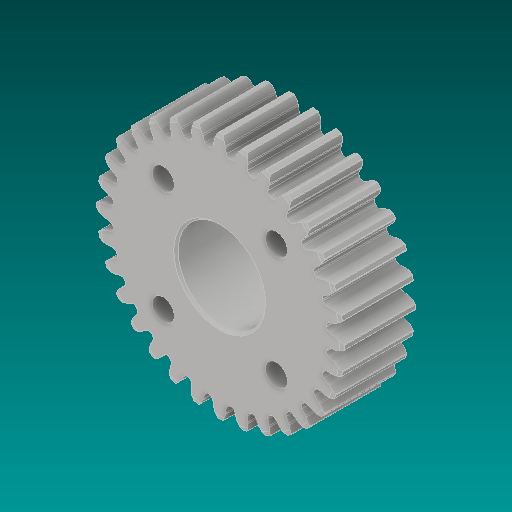
# Autodesk Inventor part: GEABP1.0-32-10-A-12-KFC22-K3_b
Saved by Autodesk Inventor 2020 (Build 240168000, 168)
## iProperties
Created: 2022-11-01
Part Number: GEABP1.0-32-10-A-12-KFC22-K3_b
Material: Generic
Catalog Web Link: www.cadenas.de
Description: GEABM, GEABMS, GEABMT, GEABP, GEABPS, GEABPT, GEABA, GEABAS, GEABAT_body-Plastic Spur Gears - Pressure Angle 20 Degrees, Module 0.5/0.8/1.0/1.5/2.0/2.5/3.0
Vendor: MISUMI
Document SubType Name: Modeling
Designer: psAdmin
Manufacturer: MISUMI
Mass: 6.51664 g
Surface Area: 40.015 cm^2
Volume: 6.51664 cm^3
Density: 1 g/cm^3
Appearance: PSOLRGB-175-175-175
Category: PARTsolutions
Company: MISUMI
PSOL_IDENT_0: {$CADENAS_DATA/23d-libs/misumi/metric/54_spur_gears/geabms20/geabms20.prj},408 {VTYP=3D},{NB=GEABP1.
PSOL_IDENT_1: 0-32-10-A-12-KFC22-K3_b},{LINA=GEABP1.0-32-10-A-12-KFC22-K3},{NN=GEABM, GEABMS, GEABMT, GEABP, GEABP
PSOL_IDENT_2: S, GEABPT, GEABA, GEABAS, GEABAT_body},{DATE=17.10.2022 23:48:33},{GEOMDATE=14.09.2022 05:11:00},{VE
PSOL_IDENT_3: RSION=},{LINEID=30},{WBVAR=MATSG,MATCR,NT,B,TS,PS,ALT1,ALT2,TPC,ALT11,ALT10,BS,ALT3,Z,J,ALT4,Q,R,S,T
PSOL_IDENT_4: ,ALT5,LFC,LTC,MALT5,ALT6,KFC,KTC,K},{WBNUMERIC=NT,B,BS,Z,J,Q,R,S,T,LFC,LTC,KFC,KTC,K}  {NB=GEABP1.0-
PSOL_IDENT_5: 32-10-A-12-KFC22-K3_b},{LINA=GEABP1.0-32-10-A-12-KFC22-K3},{KT=DUMMY},{PN=GEABP1.0-32-10-A-12-KFC22-
PSOL_IDENT_6: K3},{TYPE=GEABP},{MATSG=PW},{MATSGALG='MCN','MC Nylon','PW','Polyacetal White','PB','Polyacetal Blue'
PSOL_IDENT_7: },{MATCR=},{MATCRALG='','-','S45C','1045 Carbon Steel','SUS304','304 Stainless Steel'},{MOD=1.0},{MO
PSOL_IDENT_8: D1=1.0},{NT=32},{NTALG=15,16,18,20,22,24,25,26,28,30,32,35,36,40,45,48,50,55,60,70,75,80,90,100,120}
PSOL_IDENT_9: ,{B=10},{BALG=10,15},{TS=A},{TSALG='A','A','B','B'},{TSPN=-A},{PS=12},{PSALG='10','10','11','11','12'
PSOL_IDENT_10: ,'12','13','13','14','14','15','15','16','16','17','17','18','18'},{PSCRL='10','10','11','11','12','
PSOL_IDENT_11: 12','13','13','14','14','15','15','16','16','17','17','18','18'},{PSCRW='10','10','12','12'},{DD=32.
PSOL_IDENT_12: 0},{DD05=16},{DD08=25.6},{DD10=32},{DD15=48},{DD20=64},{DD25=80},{DD30=96},{D=34.0},{D05=17},{D08=27
PSOL_IDENT_13: .2},{D10=34},{D15=51},{D20=68},{D25=85},{D30=102},{G=29.50},{G05=14.75},{G08=23.6},{G10=29.5},{G15=4
PSOL_IDENT_14: 4.25},{G20=59},{G25=73.75},{G30=88.5},{H=0.0},{L=0},{LL1=0},{LL2=0.0},{M=-},{M3D=0},{P=12.00},{DD1=0
PSOL_IDENT_15: },{CIFR=15},{CIFM=0},{CIFK=0},{CIFTAP=0},{ALT1=},{ALT1ALG='','Not applicable'},{ALT1PN=},{ALT2=},{AL
PSOL_IDENT_16: T2ALG='','Not applicable'},{TPC=N/A},{TPCALG='N/A'},{ALT2PN=},{KC=0},{ALT11=},{ALT11ALG='','Not appl
PSOL_IDENT_17: icable'},{ALT11PN=},{DEG=0},{ALT10=},{ALT10ALG= '','Not applicable' },{ALT10PN=},{BS=0.0},{BSALG=0},
PSOL_IDENT_18: {BSMIN=3},{BSMINALG=3.000},{BSMAX=0},{LL13D=0},{LL23D=0},{LBS=10},{ALT3=},{ALT3ALG= '','w/o Stepped
PSOL_IDENT_19: Hole','DHL','with DHL (Stepped Hole)','DHR','with DHR (Stepped Hole)' },{ALT3PN=},{ZJPN=},{ALT31=1},
PSOL_IDENT_20: {ALT32=1},{Z=0},{ZALG=0},{ZMINL=14},{ZMAXL=25},{ZMINR=14},{ZMAXR=25},{ZPN=},{J=0.0},{JALG=0},{JMIN=2
PSOL_IDENT_21: },{JMAX=0},{JPN=},{ALT4=},{ALT4ALG= '','w/o WDH (Both Ends Stepped Hole)','WDH','with WDH (Both Ends
PSOL_IDENT_22: Stepped Hole)' },{ALT4PN=},{QRSTPN=},{LB=10.000},{Q=0},{QALG=0},{QMIN=14},{QMAX=25},{QPN=},{R=0},{R
PSOL_IDENT_23: ALG=0},{RMIN=14},{RMAX=25},{RPN=},{S=0},{SALG=0},{SMIN=3},{SMAX=4},{SPN=},{T=0},{TALG=0},{TMIN=3},{T
PSOL_IDENT_24: MAX=0},{TPN=},{ALT5=},{ALT5ALG= '','w/o Side Slotted Hole','LFC','with LFC (Side Slotted Hole)','LTC'
PSOL_IDENT_25: ,'with LTC (Side Slotted Hole)' },{LFC=0},{LFCALG=0},{LTC=0},{LTCALG=0},{LPCDMIN=20},{LPCDMAX=22},{L
PSOL_IDENT_26: CMAX=25},{MALT5=N/A},{MALT5ALG= 'N/A' },{LCMAX2=22},{C=0.0},{ALT5PN=},{ALT6=KFC},{ALT6ALG= '','w/o S
PSOL_IDENT_27: ide Through Hole','KFC','with KFC (Side Through Hole)','KTC','with KTC (Side Through Hole)' },{ALT6P
PSOL_IDENT_28: N=-KFC},{KFTCPN=22-K3},{KFC=22},{KFCALG=[19:22/1]},{KFCPN=22},{KTC=0},{KTCALG=[0]},{KTCPN=},{KPCDMIN
PSOL_IDENT_29: 1=19},{KPCDMAX1=-7},{KPCDMIN2=7},{KPCDMAX2=22},{K=3.0},{KALG=[3:3.5/0.5]},{KPCD=22},{KPN=-K3},{SCREW=
PSOL_IDENT_30: 0},{SCREWL=0},{AG=0},{PCD=22},{SHN=4},{SHDEG1=45},{SHDEG2=90},{PZQRDD2=12},{D1=2.8125},{D2=5.625},{D
PSOL_IDENT_31: 3=20},{D4=0.1},{D5=5.333333},{D6=4.923077},{D7=0.85},{D8=0.5},{D9=0.821781},{S1=15},{S2=0.5},{KR=15}
NB: GEABP1.0-32-10-A-12-KFC22-K3_b
NN: GEABM, GEABMS, GEABMT, GEABP, GEABPS, GEABPT, GEABA, GEABAS, GEABAT_body
NT: 32
NBSYN: $PN._b
LINA: GEABP1.0-32-10-A-12-KFC22-K3
CATALOG: Misumi
PN: GEABP1.0-32-10-A-12-KFC22-K3
MATSG: Polyacetal White
MATCR: -
MOD: 1.0
B: 10
TS: A
PS: 12
DD: 32
D: 34
G: 29.5
H: 0
L: 0
LL1: 0
LL2: 0
M: -
DD1: 0
ALT1: Not applicable
ALT2: Not applicable
TPC: N/A
ALT11: Not applicable
ALT10: Not applicable
BS: 0
ALT3: w/o Stepped Hole
Z: 0
J: 0
ALT4: w/o WDH (Both Ends Stepped Hole)
Q: 0
R: 0
S: 0
T: 0
ALT5: w/o Side Slotted Hole
LFC: 0
LTC: 0
MALT5: N/A
C: 0
ALT6: with KFC (Side Through Hole)
KFC: 22
KTC: 0
K: 3
SUPPLIER: MISUMI
ARTICLENO: GEABP1.0-32-10-A-12-KFC22-K3_b
BOMINFO: GEABP1.0-32-10-A-12-KFC22-K3
CREATOR: CADENAS GmbH
Title: GEABP1.0-32-10-A-12-KFC22-K3
Author: Cadenas PARTsolutions
Comments: Plastic Spur Gears - Pressure Angle 20 Degrees, Module 0.5/0.8/1.0/1.5/2.0/2.5/3.0
Autodesk Inventor part; units mm, degrees
ref_plane "YZ Plane" through (0, 0, 0) normal (1, 0, 0) x (0, 1, 0)
ref_plane "XZ Plane" through (0, 0, 0) normal (0, 1, 0) x (-1, 0, 0)
ref_plane "XY Plane" through (0, 0, 0) normal (0, 0, 1) x (1, 0, 0)
sketch "_____3" plane through (0, 0, 0) normal (1, 0, 0) x (0, 0, -1)
  line L0 (10, 0) -> (0, 0)
  line L1 (0, 0) -> (0, 16.5)
  line L2 (0, 16.5) -> (0.6699, 19)
  line L3 (0.6699, 19) -> (9.3301, 19)
  line L4 (9.3301, 19) -> (10, 16.5)
  line L5 (10, 16.5) -> (10, 0)
  line L6 (10, 0) -> (0, 0)
  constraints: 14 end point
revolve "Revolution1" add sketch "_____3" angle 360 about axis through (0, 0, -10) along (0, 0, -1)
sketch "_____12" plane through (0, 0, 0) normal (0, 0, 1) x (1, 0, 0)
  circle A0 centre (0, 0) radius 68
  arc A1 (-16.9975, 0.2932) -> (-16.9975, -0.2932) centre (0, 0) ccw
  arc A2 (-16.9975, -0.2932) -> (-16.9451, -0.3794) centre (-16.8975, -0.2914) ccw
  arc A3 (-16.9451, -0.3794) -> (-15.9807, -0.7851) centre (-14.4047, 4.3101) ccw
  arc A4 (-15.9807, -0.7851) -> (-15.7971, -0.8196) centre (-15.7379, 0) ccw
  arc A5 (-15.0745, -0.9267) -> (-15.7971, -0.8196) centre (-16.1556, -5.7297) ccw
  arc A6 (-14.6864, -1.3682) -> (-15.0745, -0.9267) centre (-15.1843, -1.4145) ccw
  arc A7 (-14.6864, -1.3682) -> (-14.6711, -1.5233) centre (0, 0) ccw
  arc A8 (-14.9656, -2.0319) -> (-14.6711, -1.5233) centre (-15.1685, -1.5749) ccw
  arc A9 (-15.6535, -2.278) -> (-14.9656, -2.0319) centre (-16.9629, 2.4678) ccw
  arc A10 (-15.6535, -2.278) -> (-15.8268, -2.3477) centre (-15.4355, -3.0703) ccw
  arc A11 (-15.8268, -2.3477) -> (-16.6935, -2.9338) centre (-13.2871, -7.0375) ccw
  arc A12 (-16.6935, -2.9338) -> (-16.7281, -3.0285) centre (-16.6297, -3.0107) ccw
  arc A13 (-16.7281, -3.0285) -> (-16.6137, -3.6036) centre (0, 0) ccw
  arc A14 (-16.6137, -3.6036) -> (-16.5455, -3.6779) centre (-16.516, -3.5824) ccw
  arc A15 (-16.5455, -3.6779) -> (-15.5205, -3.8877) centre (-14.9688, 1.417) ccw
  arc A16 (-15.5205, -3.8877) -> (-15.3337, -3.8858) centre (-15.4355, -3.0703) ccw
  arc A17 (-14.604, -3.8498) -> (-15.3337, -3.8858) centre (-14.7273, -8.7714) ccw
  arc A18 (-14.1373, -4.2071) -> (-14.604, -3.8498) centre (-14.6165, -4.3497) ccw
  arc A19 (-14.1373, -4.2071) -> (-14.092, -4.3562) centre (0, 0) ccw
  arc A20 (-14.2816, -4.9125) -> (-14.092, -4.3562) centre (-14.5697, -4.5039) ccw
  arc A21 (-14.9083, -5.288) -> (-14.2816, -4.9125) centre (-17.1184, -0.889) ccw
  arc A22 (-14.9083, -5.288) -> (-15.0647, -5.3902) centre (-14.5399, -6.0226) ccw
  arc A23 (-15.0647, -5.3902) -> (-15.8004, -6.1341) centre (-11.6588, -9.4944) ccw
  arc A24 (-15.8004, -6.1341) -> (-15.8158, -6.2338) centre (-15.7228, -6.1971) ccw
  arc A25 (-15.8158, -6.2338) -> (-15.5914, -6.7755) centre (0, 0) ccw
  arc A26 (-15.5914, -6.7755) -> (-15.5101, -6.8351) centre (-15.4997, -6.7356) ccw
  arc A27 (-15.5101, -6.8351) -> (-14.4638, -6.8409) centre (-14.9576, -1.5305) ccw
  arc A28 (-14.4638, -6.8409) -> (-14.281, -6.8025) centre (-14.5399, -6.0226) ccw
  arc A29 (-13.5723, -6.6249) -> (-14.281, -6.8025) centre (-12.7331, -11.476) ccw
  arc A30 (-13.0449, -6.8843) -> (-13.5723, -6.6249) centre (-13.4871, -7.1176) ccw
  arc A31 (-13.0449, -6.8843) -> (-12.9714, -7.0217) centre (0, 0) ccw
  arc A32 (-13.0488, -7.6044) -> (-12.9714, -7.0217) centre (-13.4111, -7.2598) ccw
  arc A33 (-13.5902, -8.0949) -> (-13.0488, -7.6044) centre (-16.6161, -4.2115) ccw
  arc A34 (-13.5902, -8.0949) -> (-13.7237, -8.2256) centre (-13.0856, -8.7435) ccw
  arc A35 (-13.7237, -8.2256) -> (-14.3001, -9.0988) centre (-9.5825, -11.5865) ccw
  arc A36 (-14.3001, -9.0988) -> (-14.2958, -9.1995) centre (-14.2117, -9.1454) ccw
  arc A37 (-14.2958, -9.1995) -> (-13.97, -9.687) centre (0, 0) ccw
  arc A38 (-13.97, -9.687) -> (-13.8786, -9.7296) centre (-13.8878, -9.6301) ccw
  arc A39 (-13.8786, -9.7296) -> (-12.8513, -9.5312) centre (-14.3716, -4.4191) ccw
  arc A40 (-12.8513, -9.5312) -> (-12.6795, -9.4579) centre (-13.0856, -8.7435) ccw
  arc A41 (-12.0191, -9.1455) -> (-12.6795, -9.4579) centre (-10.2496, -13.7396) ccw
  arc A42 (-11.4512, -9.2969) -> (-12.0191, -9.1455) centre (-11.8394, -9.6121) ccw
  arc A43 (-11.4512, -9.2969) -> (-11.3523, -9.4174) centre (0, 0) ccw
  arc A44 (-11.3146, -10.0039) -> (-11.3523, -9.4174) centre (-11.7371, -9.7367) ccw
  arc A45 (-11.7498, -10.5907) -> (-11.3146, -10.0039) centre (-15.4752, -7.3722) ccw
  arc A46 (-11.7498, -10.5907) -> (-11.8552, -10.7449) centre (-11.1284, -11.1284) ccw
  arc A47 (-11.8552, -10.7449) -> (-12.2503, -11.7138) centre (-7.138, -13.2334) ccw
  arc A48 (-12.2503, -11.7138) -> (-12.2263, -11.8117) centre (-12.1544, -11.7423) ccw
  arc A49 (-12.2263, -11.8117) -> (-11.8117, -12.2263) centre (0, 0) ccw
  arc A50 (-11.8117, -12.2263) -> (-11.7138, -12.2503) centre (-11.7423, -12.1544) ccw
  arc A51 (-11.7138, -12.2503) -> (-10.7449, -11.8552) centre (-13.2334, -7.138) ccw
  arc A52 (-10.7449, -11.8552) -> (-10.5907, -11.7498) centre (-11.1284, -11.1284) ccw
  arc A53 (-10.0039, -11.3146) -> (-10.5907, -11.7498) centre (-7.3722, -15.4752) ccw
  arc A54 (-9.4174, -11.3523) -> (-10.0039, -11.3146) centre (-9.7367, -11.7371) ccw
  arc A55 (-9.4174, -11.3523) -> (-9.2969, -11.4512) centre (0, 0) ccw
  arc A56 (-9.1455, -12.0191) -> (-9.2969, -11.4512) centre (-9.6121, -11.8394) ccw
  arc A57 (-9.4579, -12.6795) -> (-9.1455, -12.0191) centre (-13.7396, -10.2496) ccw
  arc A58 (-9.4579, -12.6795) -> (-9.5312, -12.8513) centre (-8.7435, -13.0856) ccw
  arc A59 (-9.5312, -12.8513) -> (-9.7296, -13.8786) centre (-4.4191, -14.3716) ccw
  arc A60 (-9.7296, -13.8786) -> (-9.687, -13.97) centre (-9.6301, -13.8878) ccw
  arc A61 (-9.687, -13.97) -> (-9.1995, -14.2958) centre (0, 0) ccw
  arc A62 (-9.1995, -14.2958) -> (-9.0988, -14.3001) centre (-9.1454, -14.2117) ccw
  arc A63 (-9.0988, -14.3001) -> (-8.2256, -13.7237) centre (-11.5865, -9.5825) ccw
  arc A64 (-8.2256, -13.7237) -> (-8.0949, -13.5902) centre (-8.7435, -13.0856) ccw
  arc A65 (-7.6044, -13.0488) -> (-8.0949, -13.5902) centre (-4.2115, -16.6161) ccw
  arc A66 (-7.0217, -12.9714) -> (-7.6044, -13.0488) centre (-7.2598, -13.4111) ccw
  arc A67 (-7.0217, -12.9714) -> (-6.8843, -13.0449) centre (0, 0) ccw
  arc A68 (-6.6249, -13.5723) -> (-6.8843, -13.0449) centre (-7.1176, -13.4871) ccw
  arc A69 (-6.8025, -14.281) -> (-6.6249, -13.5723) centre (-11.476, -12.7331) ccw
  arc A70 (-6.8025, -14.281) -> (-6.8409, -14.4638) centre (-6.0226, -14.5399) ccw
  arc A71 (-6.8409, -14.4638) -> (-6.8351, -15.5101) centre (-1.5305, -14.9576) ccw
  arc A72 (-6.8351, -15.5101) -> (-6.7755, -15.5914) centre (-6.7356, -15.4997) ccw
  arc A73 (-6.7755, -15.5914) -> (-6.2338, -15.8158) centre (0, 0) ccw
  arc A74 (-6.2338, -15.8158) -> (-6.1341, -15.8004) centre (-6.1971, -15.7228) ccw
  arc A75 (-6.1341, -15.8004) -> (-5.3902, -15.0647) centre (-9.4944, -11.6588) ccw
  arc A76 (-5.3902, -15.0647) -> (-5.288, -14.9083) centre (-6.0226, -14.5399) ccw
  arc A77 (-4.9125, -14.2816) -> (-5.288, -14.9083) centre (-0.889, -17.1184) ccw
  arc A78 (-4.3562, -14.092) -> (-4.9125, -14.2816) centre (-4.5039, -14.5697) ccw
  arc A79 (-4.3562, -14.092) -> (-4.2071, -14.1373) centre (0, 0) ccw
  arc A80 (-3.8498, -14.604) -> (-4.2071, -14.1373) centre (-4.3497, -14.6165) ccw
  arc A81 (-3.8858, -15.3337) -> (-3.8498, -14.604) centre (-8.7714, -14.7273) ccw
  arc A82 (-3.8858, -15.3337) -> (-3.8877, -15.5205) centre (-3.0703, -15.4355) ccw
  arc A83 (-3.8877, -15.5205) -> (-3.6779, -16.5455) centre (1.417, -14.9688) ccw
  arc A84 (-3.6779, -16.5455) -> (-3.6036, -16.6137) centre (-3.5824, -16.516) ccw
  arc A85 (-3.6036, -16.6137) -> (-3.0285, -16.7281) centre (0, 0) ccw
  arc A86 (-3.0285, -16.7281) -> (-2.9338, -16.6935) centre (-3.0107, -16.6297) ccw
  arc A87 (-2.9338, -16.6935) -> (-2.3477, -15.8268) centre (-7.0375, -13.2871) ccw
  arc A88 (-2.3477, -15.8268) -> (-2.278, -15.6535) centre (-3.0703, -15.4355) ccw
  arc A89 (-2.0319, -14.9656) -> (-2.278, -15.6535) centre (2.4678, -16.9629) ccw
  arc A90 (-1.5233, -14.6711) -> (-2.0319, -14.9656) centre (-1.5749, -15.1685) ccw
  arc A91 (-1.5233, -14.6711) -> (-1.3682, -14.6864) centre (0, 0) ccw
  arc A92 (-0.9267, -15.0745) -> (-1.3682, -14.6864) centre (-1.4145, -15.1843) ccw
  arc A93 (-0.8196, -15.7971) -> (-0.9267, -15.0745) centre (-5.7297, -16.1556) ccw
  arc A94 (-0.8196, -15.7971) -> (-0.7851, -15.9807) centre (0, -15.7379) ccw
  arc A95 (-0.7851, -15.9807) -> (-0.3794, -16.9451) centre (4.3101, -14.4047) ccw
  arc A96 (-0.3794, -16.9451) -> (-0.2932, -16.9975) centre (-0.2914, -16.8975) ccw
  arc A97 (-0.2932, -16.9975) -> (0.2932, -16.9975) centre (0, 0) ccw
  arc A98 (0.2932, -16.9975) -> (0.3794, -16.9451) centre (0.2914, -16.8975) ccw
  arc A99 (0.3794, -16.9451) -> (0.7851, -15.9807) centre (-4.3101, -14.4047) ccw
  arc A100 (0.7851, -15.9807) -> (0.8196, -15.7971) centre (0, -15.7379) ccw
  arc A101 (0.9267, -15.0745) -> (0.8196, -15.7971) centre (5.7297, -16.1556) ccw
  arc A102 (1.3682, -14.6864) -> (0.9267, -15.0745) centre (1.4145, -15.1843) ccw
  arc A103 (1.3682, -14.6864) -> (1.5233, -14.6711) centre (0, 0) ccw
  arc A104 (2.0319, -14.9656) -> (1.5233, -14.6711) centre (1.5749, -15.1685) ccw
  arc A105 (2.278, -15.6535) -> (2.0319, -14.9656) centre (-2.4678, -16.9629) ccw
  arc A106 (2.278, -15.6535) -> (2.3477, -15.8268) centre (3.0703, -15.4355) ccw
  arc A107 (2.3477, -15.8268) -> (2.9338, -16.6935) centre (7.0375, -13.2871) ccw
  arc A108 (2.9338, -16.6935) -> (3.0285, -16.7281) centre (3.0107, -16.6297) ccw
  arc A109 (3.0285, -16.7281) -> (3.6036, -16.6137) centre (0, 0) ccw
  arc A110 (3.6036, -16.6137) -> (3.6779, -16.5455) centre (3.5824, -16.516) ccw
  arc A111 (3.6779, -16.5455) -> (3.8877, -15.5205) centre (-1.417, -14.9688) ccw
  arc A112 (3.8877, -15.5205) -> (3.8858, -15.3337) centre (3.0703, -15.4355) ccw
  arc A113 (3.8498, -14.604) -> (3.8858, -15.3337) centre (8.7714, -14.7273) ccw
  arc A114 (4.2071, -14.1373) -> (3.8498, -14.604) centre (4.3497, -14.6165) ccw
  arc A115 (4.2071, -14.1373) -> (4.3562, -14.092) centre (0, 0) ccw
  arc A116 (4.9125, -14.2816) -> (4.3562, -14.092) centre (4.5039, -14.5697) ccw
  arc A117 (5.288, -14.9083) -> (4.9125, -14.2816) centre (0.889, -17.1184) ccw
  arc A118 (5.288, -14.9083) -> (5.3902, -15.0647) centre (6.0226, -14.5399) ccw
  arc A119 (5.3902, -15.0647) -> (6.1341, -15.8004) centre (9.4944, -11.6588) ccw
  arc A120 (6.1341, -15.8004) -> (6.2338, -15.8158) centre (6.1971, -15.7228) ccw
  arc A121 (6.2338, -15.8158) -> (6.7755, -15.5914) centre (0, 0) ccw
  arc A122 (6.7755, -15.5914) -> (6.8351, -15.5101) centre (6.7356, -15.4997) ccw
  arc A123 (6.8351, -15.5101) -> (6.8409, -14.4638) centre (1.5305, -14.9576) ccw
  arc A124 (6.8409, -14.4638) -> (6.8025, -14.281) centre (6.0226, -14.5399) ccw
  arc A125 (6.6249, -13.5723) -> (6.8025, -14.281) centre (11.476, -12.7331) ccw
  arc A126 (6.8843, -13.0449) -> (6.6249, -13.5723) centre (7.1176, -13.4871) ccw
  arc A127 (6.8843, -13.0449) -> (7.0217, -12.9714) centre (0, 0) ccw
  arc A128 (7.6044, -13.0488) -> (7.0217, -12.9714) centre (7.2598, -13.4111) ccw
  arc A129 (8.0949, -13.5902) -> (7.6044, -13.0488) centre (4.2115, -16.6161) ccw
  arc A130 (8.0949, -13.5902) -> (8.2256, -13.7237) centre (8.7435, -13.0856) ccw
  arc A131 (8.2256, -13.7237) -> (9.0988, -14.3001) centre (11.5865, -9.5825) ccw
  arc A132 (9.0988, -14.3001) -> (9.1995, -14.2958) centre (9.1454, -14.2117) ccw
  arc A133 (9.1995, -14.2958) -> (9.687, -13.97) centre (0, 0) ccw
  arc A134 (9.687, -13.97) -> (9.7296, -13.8786) centre (9.6301, -13.8878) ccw
  arc A135 (9.7296, -13.8786) -> (9.5312, -12.8513) centre (4.4191, -14.3716) ccw
  arc A136 (9.5312, -12.8513) -> (9.4579, -12.6795) centre (8.7435, -13.0856) ccw
  arc A137 (9.1455, -12.0191) -> (9.4579, -12.6795) centre (13.7396, -10.2496) ccw
  arc A138 (9.2969, -11.4512) -> (9.1455, -12.0191) centre (9.6121, -11.8394) ccw
  arc A139 (9.2969, -11.4512) -> (9.4174, -11.3523) centre (0, 0) ccw
  arc A140 (10.0039, -11.3146) -> (9.4174, -11.3523) centre (9.7367, -11.7371) ccw
  arc A141 (10.5907, -11.7498) -> (10.0039, -11.3146) centre (7.3722, -15.4752) ccw
  arc A142 (10.5907, -11.7498) -> (10.7449, -11.8552) centre (11.1284, -11.1284) ccw
  arc A143 (10.7449, -11.8552) -> (11.7138, -12.2503) centre (13.2334, -7.138) ccw
  arc A144 (11.7138, -12.2503) -> (11.8117, -12.2263) centre (11.7423, -12.1544) ccw
  arc A145 (11.8117, -12.2263) -> (12.2263, -11.8117) centre (0, 0) ccw
  arc A146 (12.2263, -11.8117) -> (12.2503, -11.7138) centre (12.1544, -11.7423) ccw
  arc A147 (12.2503, -11.7138) -> (11.8552, -10.7449) centre (7.138, -13.2334) ccw
  arc A148 (11.8552, -10.7449) -> (11.7498, -10.5907) centre (11.1284, -11.1284) ccw
  arc A149 (11.3146, -10.0039) -> (11.7498, -10.5907) centre (15.4752, -7.3722) ccw
  arc A150 (11.3523, -9.4174) -> (11.3146, -10.0039) centre (11.7371, -9.7367) ccw
  arc A151 (11.3523, -9.4174) -> (11.4512, -9.2969) centre (0, 0) ccw
  arc A152 (12.0191, -9.1455) -> (11.4512, -9.2969) centre (11.8394, -9.6121) ccw
  arc A153 (12.6795, -9.4579) -> (12.0191, -9.1455) centre (10.2496, -13.7396) ccw
  arc A154 (12.6795, -9.4579) -> (12.8513, -9.5312) centre (13.0856, -8.7435) ccw
  arc A155 (12.8513, -9.5312) -> (13.8786, -9.7296) centre (14.3716, -4.4191) ccw
  arc A156 (13.8786, -9.7296) -> (13.97, -9.687) centre (13.8878, -9.6301) ccw
  arc A157 (13.97, -9.687) -> (14.2958, -9.1995) centre (0, 0) ccw
  arc A158 (14.2958, -9.1995) -> (14.3001, -9.0988) centre (14.2117, -9.1454) ccw
  arc A159 (14.3001, -9.0988) -> (13.7237, -8.2256) centre (9.5825, -11.5865) ccw
  arc A160 (13.7237, -8.2256) -> (13.5902, -8.0949) centre (13.0856, -8.7435) ccw
  arc A161 (13.0488, -7.6044) -> (13.5902, -8.0949) centre (16.6161, -4.2115) ccw
  arc A162 (12.9714, -7.0217) -> (13.0488, -7.6044) centre (13.4111, -7.2598) ccw
  arc A163 (12.9714, -7.0217) -> (13.0449, -6.8843) centre (0, 0) ccw
  arc A164 (13.5723, -6.6249) -> (13.0449, -6.8843) centre (13.4871, -7.1176) ccw
  arc A165 (14.281, -6.8025) -> (13.5723, -6.6249) centre (12.7331, -11.476) ccw
  arc A166 (14.281, -6.8025) -> (14.4638, -6.8409) centre (14.5399, -6.0226) ccw
  arc A167 (14.4638, -6.8409) -> (15.5101, -6.8351) centre (14.9576, -1.5305) ccw
  arc A168 (15.5101, -6.8351) -> (15.5914, -6.7755) centre (15.4997, -6.7356) ccw
  arc A169 (15.5914, -6.7755) -> (15.8158, -6.2338) centre (0, 0) ccw
  arc A170 (15.8158, -6.2338) -> (15.8004, -6.1341) centre (15.7228, -6.1971) ccw
  arc A171 (15.8004, -6.1341) -> (15.0647, -5.3902) centre (11.6588, -9.4944) ccw
  arc A172 (15.0647, -5.3902) -> (14.9083, -5.288) centre (14.5399, -6.0226) ccw
  arc A173 (14.2816, -4.9125) -> (14.9083, -5.288) centre (17.1184, -0.889) ccw
  arc A174 (14.092, -4.3562) -> (14.2816, -4.9125) centre (14.5697, -4.5039) ccw
  arc A175 (14.092, -4.3562) -> (14.1373, -4.2071) centre (0, 0) ccw
  arc A176 (14.604, -3.8498) -> (14.1373, -4.2071) centre (14.6165, -4.3497) ccw
  arc A177 (15.3337, -3.8858) -> (14.604, -3.8498) centre (14.7273, -8.7714) ccw
  arc A178 (15.3337, -3.8858) -> (15.5205, -3.8877) centre (15.4355, -3.0703) ccw
  arc A179 (15.5205, -3.8877) -> (16.5455, -3.6779) centre (14.9688, 1.417) ccw
  arc A180 (16.5455, -3.6779) -> (16.6137, -3.6036) centre (16.516, -3.5824) ccw
  arc A181 (16.6137, -3.6036) -> (16.7281, -3.0285) centre (0, 0) ccw
  arc A182 (16.7281, -3.0285) -> (16.6935, -2.9338) centre (16.6297, -3.0107) ccw
  arc A183 (16.6935, -2.9338) -> (15.8268, -2.3477) centre (13.2871, -7.0375) ccw
  arc A184 (15.8268, -2.3477) -> (15.6535, -2.278) centre (15.4355, -3.0703) ccw
  arc A185 (14.9656, -2.0319) -> (15.6535, -2.278) centre (16.9629, 2.4678) ccw
  arc A186 (14.6711, -1.5233) -> (14.9656, -2.0319) centre (15.1685, -1.5749) ccw
  arc A187 (14.6711, -1.5233) -> (14.6864, -1.3682) centre (0, 0) ccw
  arc A188 (15.0745, -0.9267) -> (14.6864, -1.3682) centre (15.1843, -1.4145) ccw
  arc A189 (15.7971, -0.8196) -> (15.0745, -0.9267) centre (16.1556, -5.7297) ccw
  arc A190 (15.7971, -0.8196) -> (15.9807, -0.7851) centre (15.7379, 0) ccw
  arc A191 (15.9807, -0.7851) -> (16.9451, -0.3794) centre (14.4047, 4.3101) ccw
  arc A192 (16.9451, -0.3794) -> (16.9975, -0.2932) centre (16.8975, -0.2914) ccw
  arc A193 (16.9975, -0.2932) -> (16.9975, 0.2932) centre (0, 0) ccw
  arc A194 (16.9975, 0.2932) -> (16.9451, 0.3794) centre (16.8975, 0.2914) ccw
  arc A195 (16.9451, 0.3794) -> (15.9807, 0.7851) centre (14.4047, -4.3101) ccw
  arc A196 (15.9807, 0.7851) -> (15.7971, 0.8196) centre (15.7379, 0) ccw
  arc A197 (15.0745, 0.9267) -> (15.7971, 0.8196) centre (16.1556, 5.7297) ccw
  arc A198 (14.6864, 1.3682) -> (15.0745, 0.9267) centre (15.1843, 1.4145) ccw
  arc A199 (14.6864, 1.3682) -> (14.6711, 1.5233) centre (0, 0) ccw
  arc A200 (14.9656, 2.0319) -> (14.6711, 1.5233) centre (15.1685, 1.5749) ccw
  arc A201 (15.6535, 2.278) -> (14.9656, 2.0319) centre (16.9629, -2.4678) ccw
  arc A202 (15.6535, 2.278) -> (15.8268, 2.3477) centre (15.4355, 3.0703) ccw
  arc A203 (15.8268, 2.3477) -> (16.6935, 2.9338) centre (13.2871, 7.0375) ccw
  arc A204 (16.6935, 2.9338) -> (16.7281, 3.0285) centre (16.6297, 3.0107) ccw
  arc A205 (16.7281, 3.0285) -> (16.6137, 3.6036) centre (0, 0) ccw
  arc A206 (16.6137, 3.6036) -> (16.5455, 3.6779) centre (16.516, 3.5824) ccw
  arc A207 (16.5455, 3.6779) -> (15.5205, 3.8877) centre (14.9688, -1.417) ccw
  arc A208 (15.5205, 3.8877) -> (15.3337, 3.8858) centre (15.4355, 3.0703) ccw
  arc A209 (14.604, 3.8498) -> (15.3337, 3.8858) centre (14.7273, 8.7714) ccw
  arc A210 (14.1373, 4.2071) -> (14.604, 3.8498) centre (14.6165, 4.3497) ccw
  arc A211 (14.1373, 4.2071) -> (14.092, 4.3562) centre (0, 0) ccw
  arc A212 (14.2816, 4.9125) -> (14.092, 4.3562) centre (14.5697, 4.5039) ccw
  arc A213 (14.9083, 5.288) -> (14.2816, 4.9125) centre (17.1184, 0.889) ccw
  arc A214 (14.9083, 5.288) -> (15.0647, 5.3902) centre (14.5399, 6.0226) ccw
  arc A215 (15.0647, 5.3902) -> (15.8004, 6.1341) centre (11.6588, 9.4944) ccw
  arc A216 (15.8004, 6.1341) -> (15.8158, 6.2338) centre (15.7228, 6.1971) ccw
  arc A217 (15.8158, 6.2338) -> (15.5914, 6.7755) centre (0, 0) ccw
  arc A218 (15.5914, 6.7755) -> (15.5101, 6.8351) centre (15.4997, 6.7356) ccw
  arc A219 (15.5101, 6.8351) -> (14.4638, 6.8409) centre (14.9576, 1.5305) ccw
  arc A220 (14.4638, 6.8409) -> (14.281, 6.8025) centre (14.5399, 6.0226) ccw
  arc A221 (13.5723, 6.6249) -> (14.281, 6.8025) centre (12.7331, 11.476) ccw
  arc A222 (13.0449, 6.8843) -> (13.5723, 6.6249) centre (13.4871, 7.1176) ccw
  arc A223 (13.0449, 6.8843) -> (12.9714, 7.0217) centre (0, 0) ccw
  arc A224 (13.0488, 7.6044) -> (12.9714, 7.0217) centre (13.4111, 7.2598) ccw
  arc A225 (13.5902, 8.0949) -> (13.0488, 7.6044) centre (16.6161, 4.2115) ccw
  arc A226 (13.5902, 8.0949) -> (13.7237, 8.2256) centre (13.0856, 8.7435) ccw
  arc A227 (13.7237, 8.2256) -> (14.3001, 9.0988) centre (9.5825, 11.5865) ccw
  arc A228 (14.3001, 9.0988) -> (14.2958, 9.1995) centre (14.2117, 9.1454) ccw
  arc A229 (14.2958, 9.1995) -> (13.97, 9.687) centre (0, 0) ccw
  arc A230 (13.97, 9.687) -> (13.8786, 9.7296) centre (13.8878, 9.6301) ccw
  arc A231 (13.8786, 9.7296) -> (12.8513, 9.5312) centre (14.3716, 4.4191) ccw
  arc A232 (12.8513, 9.5312) -> (12.6795, 9.4579) centre (13.0856, 8.7435) ccw
  arc A233 (12.0191, 9.1455) -> (12.6795, 9.4579) centre (10.2496, 13.7396) ccw
  arc A234 (11.4512, 9.2969) -> (12.0191, 9.1455) centre (11.8394, 9.6121) ccw
  arc A235 (11.4512, 9.2969) -> (11.3523, 9.4174) centre (0, 0) ccw
  arc A236 (11.3146, 10.0039) -> (11.3523, 9.4174) centre (11.7371, 9.7367) ccw
  arc A237 (11.7498, 10.5907) -> (11.3146, 10.0039) centre (15.4752, 7.3722) ccw
  arc A238 (11.7498, 10.5907) -> (11.8552, 10.7449) centre (11.1284, 11.1284) ccw
  arc A239 (11.8552, 10.7449) -> (12.2503, 11.7138) centre (7.138, 13.2334) ccw
  arc A240 (12.2503, 11.7138) -> (12.2263, 11.8117) centre (12.1544, 11.7423) ccw
  arc A241 (12.2263, 11.8117) -> (11.8117, 12.2263) centre (0, 0) ccw
  arc A242 (11.8117, 12.2263) -> (11.7138, 12.2503) centre (11.7423, 12.1544) ccw
  arc A243 (11.7138, 12.2503) -> (10.7449, 11.8552) centre (13.2334, 7.138) ccw
  arc A244 (10.7449, 11.8552) -> (10.5907, 11.7498) centre (11.1284, 11.1284) ccw
  arc A245 (10.0039, 11.3146) -> (10.5907, 11.7498) centre (7.3722, 15.4752) ccw
  arc A246 (9.4174, 11.3523) -> (10.0039, 11.3146) centre (9.7367, 11.7371) ccw
  arc A247 (9.4174, 11.3523) -> (9.2969, 11.4512) centre (0, 0) ccw
  arc A248 (9.1455, 12.0191) -> (9.2969, 11.4512) centre (9.6121, 11.8394) ccw
  arc A249 (9.4579, 12.6795) -> (9.1455, 12.0191) centre (13.7396, 10.2496) ccw
  arc A250 (9.4579, 12.6795) -> (9.5312, 12.8513) centre (8.7435, 13.0856) ccw
  arc A251 (9.5312, 12.8513) -> (9.7296, 13.8786) centre (4.4191, 14.3716) ccw
  arc A252 (9.7296, 13.8786) -> (9.687, 13.97) centre (9.6301, 13.8878) ccw
  arc A253 (9.687, 13.97) -> (9.1995, 14.2958) centre (0, 0) ccw
  arc A254 (9.1995, 14.2958) -> (9.0988, 14.3001) centre (9.1454, 14.2117) ccw
  arc A255 (9.0988, 14.3001) -> (8.2256, 13.7237) centre (11.5865, 9.5825) ccw
  arc A256 (8.2256, 13.7237) -> (8.0949, 13.5902) centre (8.7435, 13.0856) ccw
  arc A257 (7.6044, 13.0488) -> (8.0949, 13.5902) centre (4.2115, 16.6161) ccw
  arc A258 (7.0217, 12.9714) -> (7.6044, 13.0488) centre (7.2598, 13.4111) ccw
  arc A259 (7.0217, 12.9714) -> (6.8843, 13.0449) centre (0, 0) ccw
  arc A260 (6.6249, 13.5723) -> (6.8843, 13.0449) centre (7.1176, 13.4871) ccw
  arc A261 (6.8025, 14.281) -> (6.6249, 13.5723) centre (11.476, 12.7331) ccw
  arc A262 (6.8025, 14.281) -> (6.8409, 14.4638) centre (6.0226, 14.5399) ccw
  arc A263 (6.8409, 14.4638) -> (6.8351, 15.5101) centre (1.5305, 14.9576) ccw
  arc A264 (6.8351, 15.5101) -> (6.7755, 15.5914) centre (6.7356, 15.4997) ccw
  arc A265 (6.7755, 15.5914) -> (6.2338, 15.8158) centre (0, 0) ccw
  arc A266 (6.2338, 15.8158) -> (6.1341, 15.8004) centre (6.1971, 15.7228) ccw
  arc A267 (6.1341, 15.8004) -> (5.3902, 15.0647) centre (9.4944, 11.6588) ccw
  arc A268 (5.3902, 15.0647) -> (5.288, 14.9083) centre (6.0226, 14.5399) ccw
  arc A269 (4.9125, 14.2816) -> (5.288, 14.9083) centre (0.889, 17.1184) ccw
  arc A270 (4.3562, 14.092) -> (4.9125, 14.2816) centre (4.5039, 14.5697) ccw
  arc A271 (4.3562, 14.092) -> (4.2071, 14.1373) centre (0, 0) ccw
  arc A272 (3.8498, 14.604) -> (4.2071, 14.1373) centre (4.3497, 14.6165) ccw
  arc A273 (3.8858, 15.3337) -> (3.8498, 14.604) centre (8.7714, 14.7273) ccw
  arc A274 (3.8858, 15.3337) -> (3.8877, 15.5205) centre (3.0703, 15.4355) ccw
  arc A275 (3.8877, 15.5205) -> (3.6779, 16.5455) centre (-1.417, 14.9688) ccw
  arc A276 (3.6779, 16.5455) -> (3.6036, 16.6137) centre (3.5824, 16.516) ccw
  arc A277 (3.6036, 16.6137) -> (3.0285, 16.7281) centre (0, 0) ccw
  arc A278 (3.0285, 16.7281) -> (2.9338, 16.6935) centre (3.0107, 16.6297) ccw
  arc A279 (2.9338, 16.6935) -> (2.3477, 15.8268) centre (7.0375, 13.2871) ccw
  arc A280 (2.3477, 15.8268) -> (2.278, 15.6535) centre (3.0703, 15.4355) ccw
  arc A281 (2.0319, 14.9656) -> (2.278, 15.6535) centre (-2.4678, 16.9629) ccw
  arc A282 (1.5233, 14.6711) -> (2.0319, 14.9656) centre (1.5749, 15.1685) ccw
  arc A283 (1.5233, 14.6711) -> (1.3682, 14.6864) centre (0, 0) ccw
  arc A284 (0.9267, 15.0745) -> (1.3682, 14.6864) centre (1.4145, 15.1843) ccw
  arc A285 (0.8196, 15.7971) -> (0.9267, 15.0745) centre (5.7297, 16.1556) ccw
  arc A286 (0.8196, 15.7971) -> (0.7851, 15.9807) centre (0, 15.7379) ccw
  arc A287 (0.7851, 15.9807) -> (0.3794, 16.9451) centre (-4.3101, 14.4047) ccw
  arc A288 (0.3794, 16.9451) -> (0.2932, 16.9975) centre (0.2914, 16.8975) ccw
  arc A289 (0.2932, 16.9975) -> (-0.2932, 16.9975) centre (0, 0) ccw
  arc A290 (-0.2932, 16.9975) -> (-0.3794, 16.9451) centre (-0.2914, 16.8975) ccw
  arc A291 (-0.3794, 16.9451) -> (-0.7851, 15.9807) centre (4.3101, 14.4047) ccw
  arc A292 (-0.7851, 15.9807) -> (-0.8196, 15.7971) centre (0, 15.7379) ccw
  arc A293 (-0.9267, 15.0745) -> (-0.8196, 15.7971) centre (-5.7297, 16.1556) ccw
  arc A294 (-1.3682, 14.6864) -> (-0.9267, 15.0745) centre (-1.4145, 15.1843) ccw
  arc A295 (-1.3682, 14.6864) -> (-1.5233, 14.6711) centre (0, 0) ccw
  arc A296 (-2.0319, 14.9656) -> (-1.5233, 14.6711) centre (-1.5749, 15.1685) ccw
  arc A297 (-2.278, 15.6535) -> (-2.0319, 14.9656) centre (2.4678, 16.9629) ccw
  arc A298 (-2.278, 15.6535) -> (-2.3477, 15.8268) centre (-3.0703, 15.4355) ccw
  arc A299 (-2.3477, 15.8268) -> (-2.9338, 16.6935) centre (-7.0375, 13.2871) ccw
  arc A300 (-2.9338, 16.6935) -> (-3.0285, 16.7281) centre (-3.0107, 16.6297) ccw
  arc A301 (-3.0285, 16.7281) -> (-3.6036, 16.6137) centre (0, 0) ccw
  arc A302 (-3.6036, 16.6137) -> (-3.6779, 16.5455) centre (-3.5824, 16.516) ccw
  arc A303 (-3.6779, 16.5455) -> (-3.8877, 15.5205) centre (1.417, 14.9688) ccw
  arc A304 (-3.8877, 15.5205) -> (-3.8858, 15.3337) centre (-3.0703, 15.4355) ccw
  arc A305 (-3.8498, 14.604) -> (-3.8858, 15.3337) centre (-8.7714, 14.7273) ccw
  arc A306 (-4.2071, 14.1373) -> (-3.8498, 14.604) centre (-4.3497, 14.6165) ccw
  arc A307 (-4.2071, 14.1373) -> (-4.3562, 14.092) centre (0, 0) ccw
  arc A308 (-4.9125, 14.2816) -> (-4.3562, 14.092) centre (-4.5039, 14.5697) ccw
  arc A309 (-5.288, 14.9083) -> (-4.9125, 14.2816) centre (-0.889, 17.1184) ccw
  arc A310 (-5.288, 14.9083) -> (-5.3902, 15.0647) centre (-6.0226, 14.5399) ccw
  arc A311 (-5.3902, 15.0647) -> (-6.1341, 15.8004) centre (-9.4944, 11.6588) ccw
  arc A312 (-6.1341, 15.8004) -> (-6.2338, 15.8158) centre (-6.1971, 15.7228) ccw
  arc A313 (-6.2338, 15.8158) -> (-6.7755, 15.5914) centre (0, 0) ccw
  arc A314 (-6.7755, 15.5914) -> (-6.8351, 15.5101) centre (-6.7356, 15.4997) ccw
  arc A315 (-6.8351, 15.5101) -> (-6.8409, 14.4638) centre (-1.5305, 14.9576) ccw
  arc A316 (-6.8409, 14.4638) -> (-6.8025, 14.281) centre (-6.0226, 14.5399) ccw
  arc A317 (-6.6249, 13.5723) -> (-6.8025, 14.281) centre (-11.476, 12.7331) ccw
  arc A318 (-6.8843, 13.0449) -> (-6.6249, 13.5723) centre (-7.1176, 13.4871) ccw
  arc A319 (-6.8843, 13.0449) -> (-7.0217, 12.9714) centre (0, 0) ccw
  arc A320 (-7.6044, 13.0488) -> (-7.0217, 12.9714) centre (-7.2598, 13.4111) ccw
  arc A321 (-8.0949, 13.5902) -> (-7.6044, 13.0488) centre (-4.2115, 16.6161) ccw
  arc A322 (-8.0949, 13.5902) -> (-8.2256, 13.7237) centre (-8.7435, 13.0856) ccw
  arc A323 (-8.2256, 13.7237) -> (-9.0988, 14.3001) centre (-11.5865, 9.5825) ccw
  arc A324 (-9.0988, 14.3001) -> (-9.1995, 14.2958) centre (-9.1454, 14.2117) ccw
  arc A325 (-9.1995, 14.2958) -> (-9.687, 13.97) centre (0, 0) ccw
  arc A326 (-9.687, 13.97) -> (-9.7296, 13.8786) centre (-9.6301, 13.8878) ccw
  arc A327 (-9.7296, 13.8786) -> (-9.5312, 12.8513) centre (-4.4191, 14.3716) ccw
  arc A328 (-9.5312, 12.8513) -> (-9.4579, 12.6795) centre (-8.7435, 13.0856) ccw
  arc A329 (-9.1455, 12.0191) -> (-9.4579, 12.6795) centre (-13.7396, 10.2496) ccw
  arc A330 (-9.2969, 11.4512) -> (-9.1455, 12.0191) centre (-9.6121, 11.8394) ccw
  arc A331 (-9.2969, 11.4512) -> (-9.4174, 11.3523) centre (0, 0) ccw
  arc A332 (-10.0039, 11.3146) -> (-9.4174, 11.3523) centre (-9.7367, 11.7371) ccw
  arc A333 (-10.5907, 11.7498) -> (-10.0039, 11.3146) centre (-7.3722, 15.4752) ccw
  arc A334 (-10.5907, 11.7498) -> (-10.7449, 11.8552) centre (-11.1284, 11.1284) ccw
  arc A335 (-10.7449, 11.8552) -> (-11.7138, 12.2503) centre (-13.2334, 7.138) ccw
  arc A336 (-11.7138, 12.2503) -> (-11.8117, 12.2263) centre (-11.7423, 12.1544) ccw
  arc A337 (-11.8117, 12.2263) -> (-12.2263, 11.8117) centre (0, 0) ccw
  arc A338 (-12.2263, 11.8117) -> (-12.2503, 11.7138) centre (-12.1544, 11.7423) ccw
  arc A339 (-12.2503, 11.7138) -> (-11.8552, 10.7449) centre (-7.138, 13.2334) ccw
  arc A340 (-11.8552, 10.7449) -> (-11.7498, 10.5907) centre (-11.1284, 11.1284) ccw
  arc A341 (-11.3146, 10.0039) -> (-11.7498, 10.5907) centre (-15.4752, 7.3722) ccw
  arc A342 (-11.3523, 9.4174) -> (-11.3146, 10.0039) centre (-11.7371, 9.7367) ccw
  arc A343 (-11.3523, 9.4174) -> (-11.4512, 9.2969) centre (0, 0) ccw
  arc A344 (-12.0191, 9.1455) -> (-11.4512, 9.2969) centre (-11.8394, 9.6121) ccw
  arc A345 (-12.6795, 9.4579) -> (-12.0191, 9.1455) centre (-10.2496, 13.7396) ccw
  arc A346 (-12.6795, 9.4579) -> (-12.8513, 9.5312) centre (-13.0856, 8.7435) ccw
  arc A347 (-12.8513, 9.5312) -> (-13.8786, 9.7296) centre (-14.3716, 4.4191) ccw
  arc A348 (-13.8786, 9.7296) -> (-13.97, 9.687) centre (-13.8878, 9.6301) ccw
  arc A349 (-13.97, 9.687) -> (-14.2958, 9.1995) centre (0, 0) ccw
  arc A350 (-14.2958, 9.1995) -> (-14.3001, 9.0988) centre (-14.2117, 9.1454) ccw
  arc A351 (-14.3001, 9.0988) -> (-13.7237, 8.2256) centre (-9.5825, 11.5865) ccw
  arc A352 (-13.7237, 8.2256) -> (-13.5902, 8.0949) centre (-13.0856, 8.7435) ccw
  arc A353 (-13.0488, 7.6044) -> (-13.5902, 8.0949) centre (-16.6161, 4.2115) ccw
  arc A354 (-12.9714, 7.0217) -> (-13.0488, 7.6044) centre (-13.4111, 7.2598) ccw
  arc A355 (-12.9714, 7.0217) -> (-13.0449, 6.8843) centre (0, 0) ccw
  arc A356 (-13.5723, 6.6249) -> (-13.0449, 6.8843) centre (-13.4871, 7.1176) ccw
  arc A357 (-14.281, 6.8025) -> (-13.5723, 6.6249) centre (-12.7331, 11.476) ccw
  arc A358 (-14.281, 6.8025) -> (-14.4638, 6.8409) centre (-14.5399, 6.0226) ccw
  arc A359 (-14.4638, 6.8409) -> (-15.5101, 6.8351) centre (-14.9576, 1.5305) ccw
  arc A360 (-15.5101, 6.8351) -> (-15.5914, 6.7755) centre (-15.4997, 6.7356) ccw
  arc A361 (-15.5914, 6.7755) -> (-15.8158, 6.2338) centre (0, 0) ccw
  arc A362 (-15.8158, 6.2338) -> (-15.8004, 6.1341) centre (-15.7228, 6.1971) ccw
  arc A363 (-15.8004, 6.1341) -> (-15.0647, 5.3902) centre (-11.6588, 9.4944) ccw
  arc A364 (-15.0647, 5.3902) -> (-14.9083, 5.288) centre (-14.5399, 6.0226) ccw
  arc A365 (-14.2816, 4.9125) -> (-14.9083, 5.288) centre (-17.1184, 0.889) ccw
  arc A366 (-14.092, 4.3562) -> (-14.2816, 4.9125) centre (-14.5697, 4.5039) ccw
  arc A367 (-14.092, 4.3562) -> (-14.1373, 4.2071) centre (0, 0) ccw
  arc A368 (-14.604, 3.8498) -> (-14.1373, 4.2071) centre (-14.6165, 4.3497) ccw
  arc A369 (-15.3337, 3.8858) -> (-14.604, 3.8498) centre (-14.7273, 8.7714) ccw
  arc A370 (-15.3337, 3.8858) -> (-15.5205, 3.8877) centre (-15.4355, 3.0703) ccw
  arc A371 (-15.5205, 3.8877) -> (-16.5455, 3.6779) centre (-14.9688, -1.417) ccw
  arc A372 (-16.5455, 3.6779) -> (-16.6137, 3.6036) centre (-16.516, 3.5824) ccw
  arc A373 (-16.6137, 3.6036) -> (-16.7281, 3.0285) centre (0, 0) ccw
  arc A374 (-16.7281, 3.0285) -> (-16.6935, 2.9338) centre (-16.6297, 3.0107) ccw
  arc A375 (-16.6935, 2.9338) -> (-15.8268, 2.3477) centre (-13.2871, 7.0375) ccw
  arc A376 (-15.8268, 2.3477) -> (-15.6535, 2.278) centre (-15.4355, 3.0703) ccw
  arc A377 (-14.9656, 2.0319) -> (-15.6535, 2.278) centre (-16.9629, -2.4678) ccw
  arc A378 (-14.6711, 1.5233) -> (-14.9656, 2.0319) centre (-15.1685, 1.5749) ccw
  arc A379 (-14.6711, 1.5233) -> (-14.6864, 1.3682) centre (0, 0) ccw
  arc A380 (-15.0745, 0.9267) -> (-14.6864, 1.3682) centre (-15.1843, 1.4145) ccw
  arc A381 (-15.7971, 0.8196) -> (-15.0745, 0.9267) centre (-16.1556, 5.7297) ccw
  arc A382 (-15.7971, 0.8196) -> (-15.9807, 0.7851) centre (-15.7379, 0) ccw
  arc A383 (-15.9807, 0.7851) -> (-16.9451, 0.3794) centre (-14.4047, -4.3101) ccw
  arc A384 (-16.9451, 0.3794) -> (-16.9975, 0.2932) centre (-16.8975, 0.2914) ccw
  constraints: 768 point on circle, 385 centre point
extrude "Extrusion1" cut sketch "_____12" against normal blind 10
sketch "Sketch3" plane through (0, 0, -10) normal (0, 0, -1) x (-0.9808, 0.1951, 0)
  point P0 (0, 0)
hole "Hole1" at (0, 0, -10) direction (0, 0, 1) diameter 12 depth 10
sketch "_____5" plane through (0, 0, 0) normal (1, 0, 0) x (0, 0, -1)
  line L0 (500, 0) -> (-500, 0)
  line L1 (9.7, 6) -> (10, 6)
  line L2 (10, 6) -> (10, 6.3)
  line L3 (10, 6.3) -> (9.7, 6)
  constraints: 8 end point
revolve "Revolution2" cut sketch "_____5" angle 360 about axis through (0, 0, -500) along (0, 0, -1)
sketch "_____13" plane through (0, 0, 0) normal (1, 0, 0) x (0, 0, -1)
  line L0 (500, 0) -> (-500, 0)
  line L1 (0, 6.3) -> (0, 6)
  line L2 (0, 6) -> (0.3, 6)
  line L3 (0.3, 6) -> (0, 6.3)
  constraints: 8 end point
revolve "Revolution3" cut sketch "_____13" angle 360 about axis through (0, 0, -500) along (0, 0, -1)
sketch "Sketch6" plane through (0, 0, -10) normal (0, 0, -1) x (-0.9808, 0.1951, 0)
  point P0 (-6.1113, 9.1462)
hole "Hole2" at (7.7782, 7.7782, -10) direction (0, 0, 1) diameter 3 depth 10
pattern_linear "Rectangular Pattern1" count 2 spacing 15.5563 along (-1, 0, 0) count 2 spacing 15.5563 along (0, -1, 0) of "Hole2"
body "Solid1"
